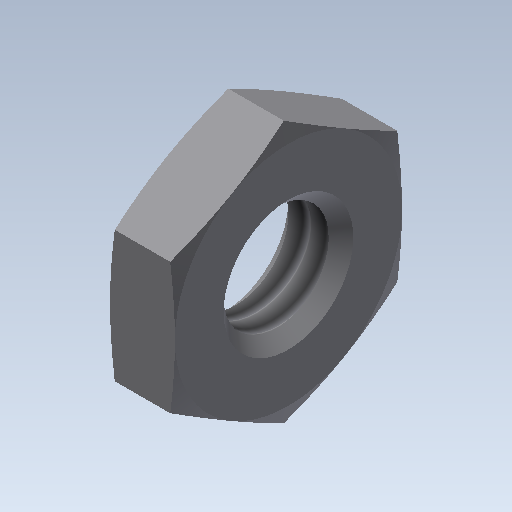
# Autodesk Inventor part: RM/8010_N2
Saved by Autodesk Inventor 2020.5 (Build 245400000, 400)
## iProperties
Created: 2018-09-27
Part Number: RM/8010_N2
Material: Generic
Catalog Web Link: www.cadenas.de
Description: Series RM/8000/M NUT2-ISO Cylinder
Vendor: IMI
Document SubType Name: Modeling
Designer: psadmin
Manufacturer: IMI
Mass: 0.0664379 g
Surface Area: 1.30945 cm^2
Volume: 0.0664379 cm^3
Density: 1 g/cm^3
Appearance: PSOLRGB-192-192-192
Category: PARTsolutions
Company: IMI
PSOL_IDENT_0: {$CADENAS_DATA\23d-libs\imi_precision\1_actuators\1_roundline_cylinders\parts\series_rm_8000_m_nut_2
PSOL_IDENT_1: .prj},175 {VTYP=3D},{NB=RM/8010_N2},{LINA=RM/8010_N2},{NN=Series RM/8000/M NUT2},{DATE=04.09.2018 05
PSOL_IDENT_2: :58:30},{GEOMDATE=04.08.2015 07:22:03},{VERSION=},{LINEID=10},{WBVAR=},{WBNUMERIC=}  {NB=RM/8010_N2}
PSOL_IDENT_3: ,{LINA=RM/8010_N2},{KT=DUMMY},{CNSORDERNO=RM/8010},{BS=010},{BSX=10},{BE=M4},{BEX=4.000},{BEP=0.700}
PSOL_IDENT_4: ,{KV=7},{KW=2}
NN: Series RM/8000/M NUT2
NT: ISO Cylinder
NB: RM/8010_N2
NBSYN: $CNSORDERNO._N2
LINA: RM/8010_N2
CNSORDERNO: RM/8010
BS: 010
BSX: 10
BE: M4
KV: 7
KW: 2
SUPPLIER: IMI
ARTICLENO: RM/8010_N2
BOMINFO: RM/8010_N2
CREATOR: CADENAS GmbH
Title: RM/8010_N2
Author: Cadenas PARTsolutions
Comments: ISO Cylinder
Autodesk Inventor part; units mm, degrees
sketch "Sketch_1" plane through (0, 0, 0) normal (0, 0, 1) x (1, 0, 0)
  line L0 (1, 0) -> (-1, 0)
  line L1 (-1, 2) -> (-0.621, 1.621)
  line L2 (-0.621, 1.621) -> (0.621, 1.621)
  line L3 (0.621, 1.621) -> (1, 2)
  line L4 (1, 2) -> (1, 3.5)
  line L5 (1, 3.5) -> (0.4824, 5.4319)
  line L6 (0.4824, 5.4319) -> (-0.4824, 5.4319)
  line L7 (-0.4824, 5.4319) -> (-1, 3.5)
  line L8 (-1, 3.5) -> (-1, 2)
  constraints: 18 end point
revolve "Revolution1" add sketch "Sketch_1" angle 360 about axis through (1, 0, 0) along (1, 0, 0)
thread "Thread1" size "M4x0.7" class "6H" standard "ISO Metric profile" full length
sketch "Sketch_2" plane through (0, 0, 0) normal (1, 0, 0) x (0, 1, 0)
  line L0 (-14, 14) -> (-14, -14)
  line L1 (-14, -14) -> (14, -14)
  line L2 (14, -14) -> (14, 14)
  line L3 (14, 14) -> (-14, 14)
  line L4 (-2.0207, 3.5) -> (-4.0415, 0)
  line L5 (-4.0415, 0) -> (-2.0207, -3.5)
  line L6 (-2.0207, -3.5) -> (2.0207, -3.5)
  line L7 (2.0207, -3.5) -> (4.0415, 0)
  line L8 (4.0415, 0) -> (2.0207, 3.5)
  line L9 (2.0207, 3.5) -> (-2.0207, 3.5)
  constraints: 20 end point
extrude "Extrusion1" cut sketch "Sketch_2" along normal mid plane 2
ref_plane "NUT_XY" through (0, 0, 0) normal (1, 0, 0) x (0, 0, -1)
ref_plane "NUT_YZ" through (0, 0, 0) normal (0, 0, -1) x (0, 1, 0)
ref_plane "NUT_ZX" through (0, 0, 0) normal (0, 1, 0) x (1, 0, 0)
body "Solid1"
